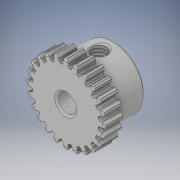
# Autodesk Inventor part: GEABP0.5-24-3-B-3_b
Saved by Autodesk Inventor 2019 (Build 230136000, 136)
## iProperties
Created: 2024-02-14
Part Number: GEABP0.5-24-3-B-3_b
Material: Generic
Catalog Web Link: www.cadenas.de
Description: GEABM, GEABMS, GEABMT, GEABP, GEABPS, GEABPT, GEABA, GEABAS, GEABAT_body-Plastic Spur Gears - Pressure Angle 20 Degrees, Module 0.5/0.8/1.0/1.5/2.0/2.5/3.0
Vendor: MISUMI
Document SubType Name: Modeling
Designer: psAdmin
Manufacturer: MISUMI
Mass: 0.648666 g
Surface Area: 6.64775 cm^2
Volume: 0.648666 cm^3
Density: 1 g/cm^3
Appearance: PSOLRGB-175-175-175
Category: PARTsolutions
Company: MISUMI
Title: GEABP0.5-24-3-B-3
Author: Cadenas PARTsolutions
Comments: Plastic Spur Gears - Pressure Angle 20 Degrees, Module 0.5/0.8/1.0/1.5/2.0/2.5/3.0
PSOL_IDENT_0: {$CADENAS_DATA/23d-libs/misumi/metric/54_spur_gears/geabms20/geabms20.prj},386 {VTYP=3D},{NB=GEABP0.
PSOL_IDENT_1: 5-24-3-B-3_b},{LINA=GEABP0.5-24-3-B-3},{NN=GEABM, GEABMS, GEABMT, GEABP, GEABPS, GEABPT, GEABA, GEAB
PSOL_IDENT_2: AS, GEABAT_body},{DATE=13.11.2023 01:03:00},{GEOMDATE=12.11.2023 05:54:16},{VERSION=},{LINEID=10},{W
PSOL_IDENT_3: BVAR=MATSG,MATCR,NT,B,TS,PS,ALT1,ALT2,TPC,ALT11,ALT10,BS,ALT3,Z,J,ALT4,Q,R,S,T,ALT5,LFC,LTC,MALT5,AL
PSOL_IDENT_4: T6,KFC,KTC,K},{WBNUMERIC=NT,B,BS,Z,J,Q,R,S,T,LFC,LTC,KFC,KTC,K}  {NB=GEABP0.5-24-3-B-3_b},{LINA=GEAB
PSOL_IDENT_5: P0.5-24-3-B-3},{KT=DUMMY},{PN=GEABP0.5-24-3-B-3},{TYPE=GEABP},{MATSG=PW},{MATSGALG='MCN','MC Nylon','
PSOL_IDENT_6: PW','Polyacetal White','PB','Polyacetal Blue'},{MATCR=},{MATCRALG='','-'},{MOD=0.5},{MOD1=0.5},{NT=2
PSOL_IDENT_7: 4},{NTALG=15,16,18,20,24,25,28,30,32,36,40,45,48,50,56,60,64,70,72,80,90,100,120},{B=3},{BALG=3,5},{
PSOL_IDENT_8: TS=B},{TSALG='B','B'},{TSPN=-B},{PS=3},{PSALG='3','3','4','4','5','5','6','6','7','7'},{PSCRL='3','3'
PSOL_IDENT_9: ,'4','4','5','5','6','6','7','7'},{PSCRW='0','0'},{DD=12.0},{DD05=12},{DD08=19.2},{DD10=24},{DD15=36
PSOL_IDENT_10: },{DD20=48},{DD25=60},{DD30=72},{D=13.0},{D05=13},{D08=20.8},{D10=26},{D15=39},{D20=52},{D25=65},{D3
PSOL_IDENT_11: 0=78},{G=10.75},{G05=10.75},{G08=17.2},{G10=21.5},{G15=32.25},{G20=43},{G25=53.75},{G30=64.5},{H=10.
PSOL_IDENT_12: 0},{L=8},{LL1=5},{LL2=2.5},{M=M3},{M3D=3},{P=3.00},{DD1=0},{CIFR=8.8},{CIFM=3},{CIFK=0},{CIFTAP=1},{
PSOL_IDENT_13: ALT1=},{ALT1ALG='','w/o Set Screw','KC90','with KC90 (Set Screw)','KC120','with KC120 (Set Screw)'},
PSOL_IDENT_14: {ALT1PN=},{ALT2=},{ALT2ALG='','w/o TPC (Tapped Hole Dimension)','TPC','with TPC (Tapped Hole Dimensi
PSOL_IDENT_15: on)'},{TPC=N/A},{TPCALG='N/A'},{ALT2PN=},{KC=0},{ALT11=},{ALT11ALG='','Not applicable'},{ALT11PN=},{
PSOL_IDENT_16: DEG=0},{ALT10=},{ALT10ALG= '','w/o BS (Boss Cut)','BS','with BS (Boss Cut)' },{ALT10PN=},{BS=0.0},{B
PSOL_IDENT_17: SALG=0},{BSMIN=6},{BSMINALG=6.000},{BSMAX=5},{LL13D=5},{LL23D=5.5},{LBS=8},{ALT3=},{ALT3ALG= '','w/o
PSOL_IDENT_18: Stepped Hole','DHR','with DHR (Stepped Hole)' },{ALT3PN=},{ZJPN=},{ALT31=0},{ALT32=1},{Z=0},{ZALG=0
PSOL_IDENT_19: },{ZMINL=5},{ZMAXL=6},{ZMINR=5},{ZMAXR=6},{ZPN=},{J=0.0},{JALG=0},{JMIN=2},{JMAX=0},{JPN=},{ALT4=},{
PSOL_IDENT_20: ALT4ALG= '','Not applicable' },{ALT4PN=},{QRSTPN=},{LB=8.000},{Q=0},{QALG=0},{QMIN=5},{QMAX=6},{QPN=
PSOL_IDENT_21: },{R=0},{RALG=0},{RMIN=5},{RMAX=6},{RPN=},{S=0},{SALG=0},{SMIN=3},{SMAX=2},{SPN=},{T=0},{TALG=0},{TM
PSOL_IDENT_22: IN=3},{TMAX=0},{TPN=},{ALT5=},{ALT5ALG= '','Not applicable' },{LFC=0},{LFCALG=0},{LTC=0},{LTCALG=0},
PSOL_IDENT_23: {LPCDMIN=11},{LPCDMAX=3},{LCMAX=6},{MALT5=N/A},{MALT5ALG= 'N/A' },{LCMAX2=3},{C=0.0},{ALT5PN=},{ALT6=
PSOL_IDENT_24: },{ALT6ALG= '','Not applicable' },{ALT6PN=},{KFTCPN=},{KFC=0},{KFCALG=[0]},{KFCPN=},{KTC=0},{KTCALG=
PSOL_IDENT_25: [0]},{KTCPN=},{KPCDMIN1=10},{KPCDMAX1=3},{KPCDMIN2=17},{KPCDMAX2=3},{K=0.0},{KALG=[0]},{KPCD=0},{KPN=
PSOL_IDENT_26: },{SCREW=3},{SCREWL=3},{AG=0},{PCD=0},{SHN=0},{SHDEG1=0},{SHDEG2=0},{PZQRDD2=3},{D1=3.75},{D2=7.5},{
PSOL_IDENT_27: D3=20},{D4=0.05},{D5=2},{D6=1.846154},{D7=0.425},{D8=0.25},{D9=0.408748},{S1=15},{S2=0.5},{KR=8.8}
NB: GEABP0.5-24-3-B-3_b
NN: GEABM, GEABMS, GEABMT, GEABP, GEABPS, GEABPT, GEABA, GEABAS, GEABAT_body
NT: 24
NBSYN: $PN._b
LINA: GEABP0.5-24-3-B-3
CATALOG: Misumi
PN: GEABP0.5-24-3-B-3
MATSG: Polyacetal White
MATCR: -
MOD: 0.5
B: 3
TS: B
PS: 3
DD: 12
D: 13
G: 10.75
H: 10
L: 8
LL1: 5
LL2: 2.5
M: M3
DD1: 0
ALT1: w/o Set Screw
ALT2: w/o TPC (Tapped Hole Dimension)
TPC: N/A
ALT11: Not applicable
ALT10: w/o BS (Boss Cut)
BS: 0
ALT3: w/o Stepped Hole
Z: 0
J: 0
ALT4: Not applicable
Q: 0
R: 0
S: 0
T: 0
ALT5: Not applicable
LFC: 0
LTC: 0
MALT5: N/A
C: 0
ALT6: Not applicable
KFC: 0
KTC: 0
K: 0
SUPPLIER: MISUMI
ARTICLENO: GEABP0.5-24-3-B-3_b
BOMINFO: GEABP0.5-24-3-B-3
CREATOR: CADENAS GmbH
Autodesk Inventor part; units mm, degrees
sketch "Sketch_2" plane through (0, 0, 0) normal (1, 0, 0) x (0, 1, 0)
  line L0 (0, -500) -> (0, 500)
  line L1 (0, 0) -> (6, 0)
  line L2 (6, 0) -> (8.5, -0.6699)
  line L3 (8.5, -0.6699) -> (8.5, -2.3301)
  line L4 (8.5, -2.3301) -> (6, -3)
  line L5 (6, -3) -> (5, -3)
  line L6 (5, -3) -> (5, -7.7)
  line L7 (5, -7.7) -> (4.7, -8)
  line L8 (4.7, -8) -> (0, -8)
  line L9 (0, -8) -> (0, 0)
  constraints: 20 end point
revolve "Revolution1" add sketch "Sketch_2" angle 360 about axis through (0, 0, -500) along (0, 0, -1)
sketch "_____12" plane through (0, 0, 0) normal (0, 0, 1) x (1, 0, 0)
  circle A0 centre (0, 0) radius 26
  arc A1 (-6.4986, 0.1346) -> (-6.4986, -0.1346) centre (0, 0) ccw
  arc A2 (-6.4986, -0.1346) -> (-6.4748, -0.1762) centre (-6.4486, -0.1336) ccw
  arc A3 (-6.4748, -0.1762) -> (-5.9872, -0.3924) centre (-5.4275, 1.5277) ccw
  arc A4 (-5.9872, -0.3924) -> (-5.8765, -0.4087) centre (-5.8728, 0) ccw
  arc A5 (-5.5335, -0.4445) -> (-5.8765, -0.4087) centre (-5.8958, -2.2548) ccw
  arc A6 (-5.3344, -0.659) -> (-5.5335, -0.4445) centre (-5.5826, -0.6897) ccw
  arc A7 (-5.3344, -0.659) -> (-5.3232, -0.7441) centre (0, 0) ccw
  arc A8 (-5.46, -1.0028) -> (-5.3232, -0.7441) centre (-5.5708, -0.7787) ccw
  arc A9 (-5.782, -1.1261) -> (-5.46, -1.0028) centre (-6.2785, 0.652) ccw
  arc A10 (-5.782, -1.1261) -> (-5.8847, -1.1705) centre (-5.6727, -1.52) ccw
  arc A11 (-5.8847, -1.1705) -> (-6.2998, -1.5056) centre (-4.8472, -2.8804) ccw
  arc A12 (-6.2998, -1.5056) -> (-6.312, -1.5519) centre (-6.2635, -1.54) ccw
  arc A13 (-6.312, -1.5519) -> (-6.2423, -1.812) centre (0, 0) ccw
  arc A14 (-6.2423, -1.812) -> (-6.2086, -1.846) centre (-6.1943, -1.7981) ccw
  arc A15 (-6.2086, -1.846) -> (-5.6816, -1.9286) centre (-5.638, 0.0709) ccw
  arc A16 (-5.6816, -1.9286) -> (-5.5704, -1.9157) centre (-5.6727, -1.52) ccw
  arc A17 (-5.2299, -1.8616) -> (-5.5704, -1.9157) centre (-5.1113, -3.7039) ccw
  arc A18 (-4.9821, -2.0172) -> (-5.2299, -1.8616) centre (-5.2138, -2.111) ccw
  arc A19 (-4.9821, -2.0172) -> (-4.9493, -2.0965) centre (0, 0) ccw
  arc A20 (-5.0144, -2.3818) -> (-4.9493, -2.0965) centre (-5.1795, -2.194) ccw
  arc A21 (-5.2935, -2.5843) -> (-5.0144, -2.3818) centre (-6.2333, -0.9952) ccw
  arc A22 (-5.2935, -2.5843) -> (-5.3812, -2.6537) centre (-5.086, -2.9364) ccw
  arc A23 (-5.3812, -2.6537) -> (-5.6954, -3.0848) centre (-3.9365, -4.0368) ccw
  arc A24 (-5.6954, -3.0848) -> (-5.6953, -3.1327) centre (-5.6515, -3.1086) ccw
  arc A25 (-5.6953, -3.1327) -> (-5.5606, -3.3659) centre (0, 0) ccw
  arc A26 (-5.5606, -3.3659) -> (-5.5192, -3.39) centre (-5.5179, -3.34) ccw
  arc A27 (-5.5192, -3.39) -> (-4.9888, -3.3334) centre (-5.4642, -1.3907) ccw
  arc A28 (-4.9888, -3.3334) -> (-4.8848, -3.2922) centre (-5.086, -2.9364) ccw
  arc A29 (-4.5699, -3.1517) -> (-4.8848, -3.2922) centre (-3.9785, -4.9006) ccw
  arc A30 (-4.2903, -3.2379) -> (-4.5699, -3.1517) centre (-4.4898, -3.3885) ccw
  arc A31 (-4.2903, -3.2379) -> (-4.238, -3.306) centre (0, 0) ccw
  arc A32 (-4.2271, -3.5985) -> (-4.238, -3.306) centre (-4.4351, -3.4598) ccw
  arc A33 (-4.4443, -3.8663) -> (-4.2271, -3.5985) centre (-5.7633, -2.5746) ccw
  arc A34 (-4.4443, -3.8663) -> (-4.511, -3.9561) centre (-4.1527, -4.1527) ccw
  arc A35 (-4.511, -3.9561) -> (-4.703, -4.4538) centre (-2.7576, -4.9181) ccw
  arc A36 (-4.703, -4.4538) -> (-4.6904, -4.5) centre (-4.6543, -4.4654) ccw
  arc A37 (-4.6904, -4.5) -> (-4.5, -4.6904) centre (0, 0) ccw
  arc A38 (-4.5, -4.6904) -> (-4.4538, -4.703) centre (-4.4654, -4.6543) ccw
  arc A39 (-4.4538, -4.703) -> (-3.9561, -4.511) centre (-4.9181, -2.7576) ccw
  arc A40 (-3.9561, -4.511) -> (-3.8663, -4.4443) centre (-4.1527, -4.1527) ccw
  arc A41 (-3.5985, -4.2271) -> (-3.8663, -4.4443) centre (-2.5746, -5.7633) ccw
  arc A42 (-3.306, -4.238) -> (-3.5985, -4.2271) centre (-3.4598, -4.4351) ccw
  arc A43 (-3.306, -4.238) -> (-3.2379, -4.2903) centre (0, 0) ccw
  arc A44 (-3.1517, -4.5699) -> (-3.2379, -4.2903) centre (-3.3885, -4.4898) ccw
  arc A45 (-3.2922, -4.8848) -> (-3.1517, -4.5699) centre (-4.9006, -3.9785) ccw
  arc A46 (-3.2922, -4.8848) -> (-3.3334, -4.9888) centre (-2.9364, -5.086) ccw
  arc A47 (-3.3334, -4.9888) -> (-3.39, -5.5192) centre (-1.3907, -5.4642) ccw
  arc A48 (-3.39, -5.5192) -> (-3.3659, -5.5606) centre (-3.34, -5.5179) ccw
  arc A49 (-3.3659, -5.5606) -> (-3.1327, -5.6953) centre (0, 0) ccw
  arc A50 (-3.1327, -5.6953) -> (-3.0848, -5.6954) centre (-3.1086, -5.6515) ccw
  arc A51 (-3.0848, -5.6954) -> (-2.6537, -5.3812) centre (-4.0368, -3.9365) ccw
  arc A52 (-2.6537, -5.3812) -> (-2.5843, -5.2935) centre (-2.9364, -5.086) ccw
  arc A53 (-2.3818, -5.0144) -> (-2.5843, -5.2935) centre (-0.9952, -6.2333) ccw
  arc A54 (-2.0965, -4.9493) -> (-2.3818, -5.0144) centre (-2.194, -5.1795) ccw
  arc A55 (-2.0965, -4.9493) -> (-2.0172, -4.9821) centre (0, 0) ccw
  arc A56 (-1.8616, -5.2299) -> (-2.0172, -4.9821) centre (-2.111, -5.2138) ccw
  arc A57 (-1.9157, -5.5704) -> (-1.8616, -5.2299) centre (-3.7039, -5.1113) ccw
  arc A58 (-1.9157, -5.5704) -> (-1.9286, -5.6816) centre (-1.52, -5.6727) ccw
  arc A59 (-1.9286, -5.6816) -> (-1.846, -6.2086) centre (0.0709, -5.638) ccw
  arc A60 (-1.846, -6.2086) -> (-1.812, -6.2423) centre (-1.7981, -6.1943) ccw
  arc A61 (-1.812, -6.2423) -> (-1.5519, -6.312) centre (0, 0) ccw
  arc A62 (-1.5519, -6.312) -> (-1.5056, -6.2998) centre (-1.54, -6.2635) ccw
  arc A63 (-1.5056, -6.2998) -> (-1.1705, -5.8847) centre (-2.8804, -4.8472) ccw
  arc A64 (-1.1705, -5.8847) -> (-1.1261, -5.782) centre (-1.52, -5.6727) ccw
  arc A65 (-1.0028, -5.46) -> (-1.1261, -5.782) centre (0.652, -6.2785) ccw
  arc A66 (-0.7441, -5.3232) -> (-1.0028, -5.46) centre (-0.7787, -5.5708) ccw
  arc A67 (-0.7441, -5.3232) -> (-0.659, -5.3344) centre (0, 0) ccw
  arc A68 (-0.4445, -5.5335) -> (-0.659, -5.3344) centre (-0.6897, -5.5826) ccw
  arc A69 (-0.4087, -5.8765) -> (-0.4445, -5.5335) centre (-2.2548, -5.8958) ccw
  arc A70 (-0.4087, -5.8765) -> (-0.3924, -5.9872) centre (0, -5.8728) ccw
  arc A71 (-0.3924, -5.9872) -> (-0.1762, -6.4748) centre (1.5277, -5.4275) ccw
  arc A72 (-0.1762, -6.4748) -> (-0.1346, -6.4986) centre (-0.1336, -6.4486) ccw
  arc A73 (-0.1346, -6.4986) -> (0.1346, -6.4986) centre (0, 0) ccw
  arc A74 (0.1346, -6.4986) -> (0.1762, -6.4748) centre (0.1336, -6.4486) ccw
  arc A75 (0.1762, -6.4748) -> (0.3924, -5.9872) centre (-1.5277, -5.4275) ccw
  arc A76 (0.3924, -5.9872) -> (0.4087, -5.8765) centre (0, -5.8728) ccw
  arc A77 (0.4445, -5.5335) -> (0.4087, -5.8765) centre (2.2548, -5.8958) ccw
  arc A78 (0.659, -5.3344) -> (0.4445, -5.5335) centre (0.6897, -5.5826) ccw
  arc A79 (0.659, -5.3344) -> (0.7441, -5.3232) centre (0, 0) ccw
  arc A80 (1.0028, -5.46) -> (0.7441, -5.3232) centre (0.7787, -5.5708) ccw
  arc A81 (1.1261, -5.782) -> (1.0028, -5.46) centre (-0.652, -6.2785) ccw
  arc A82 (1.1261, -5.782) -> (1.1705, -5.8847) centre (1.52, -5.6727) ccw
  arc A83 (1.1705, -5.8847) -> (1.5056, -6.2998) centre (2.8804, -4.8472) ccw
  arc A84 (1.5056, -6.2998) -> (1.5519, -6.312) centre (1.54, -6.2635) ccw
  arc A85 (1.5519, -6.312) -> (1.812, -6.2423) centre (0, 0) ccw
  arc A86 (1.812, -6.2423) -> (1.846, -6.2086) centre (1.7981, -6.1943) ccw
  arc A87 (1.846, -6.2086) -> (1.9286, -5.6816) centre (-0.0709, -5.638) ccw
  arc A88 (1.9286, -5.6816) -> (1.9157, -5.5704) centre (1.52, -5.6727) ccw
  arc A89 (1.8616, -5.2299) -> (1.9157, -5.5704) centre (3.7039, -5.1113) ccw
  arc A90 (2.0172, -4.9821) -> (1.8616, -5.2299) centre (2.111, -5.2138) ccw
  arc A91 (2.0172, -4.9821) -> (2.0965, -4.9493) centre (0, 0) ccw
  arc A92 (2.3818, -5.0144) -> (2.0965, -4.9493) centre (2.194, -5.1795) ccw
  arc A93 (2.5843, -5.2935) -> (2.3818, -5.0144) centre (0.9952, -6.2333) ccw
  arc A94 (2.5843, -5.2935) -> (2.6537, -5.3812) centre (2.9364, -5.086) ccw
  arc A95 (2.6537, -5.3812) -> (3.0848, -5.6954) centre (4.0368, -3.9365) ccw
  arc A96 (3.0848, -5.6954) -> (3.1327, -5.6953) centre (3.1086, -5.6515) ccw
  arc A97 (3.1327, -5.6953) -> (3.3659, -5.5606) centre (0, 0) ccw
  arc A98 (3.3659, -5.5606) -> (3.39, -5.5192) centre (3.34, -5.5179) ccw
  arc A99 (3.39, -5.5192) -> (3.3334, -4.9888) centre (1.3907, -5.4642) ccw
  arc A100 (3.3334, -4.9888) -> (3.2922, -4.8848) centre (2.9364, -5.086) ccw
  arc A101 (3.1517, -4.5699) -> (3.2922, -4.8848) centre (4.9006, -3.9785) ccw
  arc A102 (3.2379, -4.2903) -> (3.1517, -4.5699) centre (3.3885, -4.4898) ccw
  arc A103 (3.2379, -4.2903) -> (3.306, -4.238) centre (0, 0) ccw
  arc A104 (3.5985, -4.2271) -> (3.306, -4.238) centre (3.4598, -4.4351) ccw
  arc A105 (3.8663, -4.4443) -> (3.5985, -4.2271) centre (2.5746, -5.7633) ccw
  arc A106 (3.8663, -4.4443) -> (3.9561, -4.511) centre (4.1527, -4.1527) ccw
  arc A107 (3.9561, -4.511) -> (4.4538, -4.703) centre (4.9181, -2.7576) ccw
  arc A108 (4.4538, -4.703) -> (4.5, -4.6904) centre (4.4654, -4.6543) ccw
  arc A109 (4.5, -4.6904) -> (4.6904, -4.5) centre (0, 0) ccw
  arc A110 (4.6904, -4.5) -> (4.703, -4.4538) centre (4.6543, -4.4654) ccw
  arc A111 (4.703, -4.4538) -> (4.511, -3.9561) centre (2.7576, -4.9181) ccw
  arc A112 (4.511, -3.9561) -> (4.4443, -3.8663) centre (4.1527, -4.1527) ccw
  arc A113 (4.2271, -3.5985) -> (4.4443, -3.8663) centre (5.7633, -2.5746) ccw
  arc A114 (4.238, -3.306) -> (4.2271, -3.5985) centre (4.4351, -3.4598) ccw
  arc A115 (4.238, -3.306) -> (4.2903, -3.2379) centre (0, 0) ccw
  arc A116 (4.5699, -3.1517) -> (4.2903, -3.2379) centre (4.4898, -3.3885) ccw
  arc A117 (4.8848, -3.2922) -> (4.5699, -3.1517) centre (3.9785, -4.9006) ccw
  arc A118 (4.8848, -3.2922) -> (4.9888, -3.3334) centre (5.086, -2.9364) ccw
  arc A119 (4.9888, -3.3334) -> (5.5192, -3.39) centre (5.4642, -1.3907) ccw
  arc A120 (5.5192, -3.39) -> (5.5606, -3.3659) centre (5.5179, -3.34) ccw
  arc A121 (5.5606, -3.3659) -> (5.6953, -3.1327) centre (0, 0) ccw
  arc A122 (5.6953, -3.1327) -> (5.6954, -3.0848) centre (5.6515, -3.1086) ccw
  arc A123 (5.6954, -3.0848) -> (5.3812, -2.6537) centre (3.9365, -4.0368) ccw
  arc A124 (5.3812, -2.6537) -> (5.2935, -2.5843) centre (5.086, -2.9364) ccw
  arc A125 (5.0144, -2.3818) -> (5.2935, -2.5843) centre (6.2333, -0.9952) ccw
  arc A126 (4.9493, -2.0965) -> (5.0144, -2.3818) centre (5.1795, -2.194) ccw
  arc A127 (4.9493, -2.0965) -> (4.9821, -2.0172) centre (0, 0) ccw
  arc A128 (5.2299, -1.8616) -> (4.9821, -2.0172) centre (5.2138, -2.111) ccw
  arc A129 (5.5704, -1.9157) -> (5.2299, -1.8616) centre (5.1113, -3.7039) ccw
  arc A130 (5.5704, -1.9157) -> (5.6816, -1.9286) centre (5.6727, -1.52) ccw
  arc A131 (5.6816, -1.9286) -> (6.2086, -1.846) centre (5.638, 0.0709) ccw
  arc A132 (6.2086, -1.846) -> (6.2423, -1.812) centre (6.1943, -1.7981) ccw
  arc A133 (6.2423, -1.812) -> (6.312, -1.5519) centre (0, 0) ccw
  arc A134 (6.312, -1.5519) -> (6.2998, -1.5056) centre (6.2635, -1.54) ccw
  arc A135 (6.2998, -1.5056) -> (5.8847, -1.1705) centre (4.8472, -2.8804) ccw
  arc A136 (5.8847, -1.1705) -> (5.782, -1.1261) centre (5.6727, -1.52) ccw
  arc A137 (5.46, -1.0028) -> (5.782, -1.1261) centre (6.2785, 0.652) ccw
  arc A138 (5.3232, -0.7441) -> (5.46, -1.0028) centre (5.5708, -0.7787) ccw
  arc A139 (5.3232, -0.7441) -> (5.3344, -0.659) centre (0, 0) ccw
  arc A140 (5.5335, -0.4445) -> (5.3344, -0.659) centre (5.5826, -0.6897) ccw
  arc A141 (5.8765, -0.4087) -> (5.5335, -0.4445) centre (5.8958, -2.2548) ccw
  arc A142 (5.8765, -0.4087) -> (5.9872, -0.3924) centre (5.8728, 0) ccw
  arc A143 (5.9872, -0.3924) -> (6.4748, -0.1762) centre (5.4275, 1.5277) ccw
  arc A144 (6.4748, -0.1762) -> (6.4986, -0.1346) centre (6.4486, -0.1336) ccw
  arc A145 (6.4986, -0.1346) -> (6.4986, 0.1346) centre (0, 0) ccw
  arc A146 (6.4986, 0.1346) -> (6.4748, 0.1762) centre (6.4486, 0.1336) ccw
  arc A147 (6.4748, 0.1762) -> (5.9872, 0.3924) centre (5.4275, -1.5277) ccw
  arc A148 (5.9872, 0.3924) -> (5.8765, 0.4087) centre (5.8728, 0) ccw
  arc A149 (5.5335, 0.4445) -> (5.8765, 0.4087) centre (5.8958, 2.2548) ccw
  arc A150 (5.3344, 0.659) -> (5.5335, 0.4445) centre (5.5826, 0.6897) ccw
  arc A151 (5.3344, 0.659) -> (5.3232, 0.7441) centre (0, 0) ccw
  arc A152 (5.46, 1.0028) -> (5.3232, 0.7441) centre (5.5708, 0.7787) ccw
  arc A153 (5.782, 1.1261) -> (5.46, 1.0028) centre (6.2785, -0.652) ccw
  arc A154 (5.782, 1.1261) -> (5.8847, 1.1705) centre (5.6727, 1.52) ccw
  arc A155 (5.8847, 1.1705) -> (6.2998, 1.5056) centre (4.8472, 2.8804) ccw
  arc A156 (6.2998, 1.5056) -> (6.312, 1.5519) centre (6.2635, 1.54) ccw
  arc A157 (6.312, 1.5519) -> (6.2423, 1.812) centre (0, 0) ccw
  arc A158 (6.2423, 1.812) -> (6.2086, 1.846) centre (6.1943, 1.7981) ccw
  arc A159 (6.2086, 1.846) -> (5.6816, 1.9286) centre (5.638, -0.0709) ccw
  arc A160 (5.6816, 1.9286) -> (5.5704, 1.9157) centre (5.6727, 1.52) ccw
  arc A161 (5.2299, 1.8616) -> (5.5704, 1.9157) centre (5.1113, 3.7039) ccw
  arc A162 (4.9821, 2.0172) -> (5.2299, 1.8616) centre (5.2138, 2.111) ccw
  arc A163 (4.9821, 2.0172) -> (4.9493, 2.0965) centre (0, 0) ccw
  arc A164 (5.0144, 2.3818) -> (4.9493, 2.0965) centre (5.1795, 2.194) ccw
  arc A165 (5.2935, 2.5843) -> (5.0144, 2.3818) centre (6.2333, 0.9952) ccw
  arc A166 (5.2935, 2.5843) -> (5.3812, 2.6537) centre (5.086, 2.9364) ccw
  arc A167 (5.3812, 2.6537) -> (5.6954, 3.0848) centre (3.9365, 4.0368) ccw
  arc A168 (5.6954, 3.0848) -> (5.6953, 3.1327) centre (5.6515, 3.1086) ccw
  arc A169 (5.6953, 3.1327) -> (5.5606, 3.3659) centre (0, 0) ccw
  arc A170 (5.5606, 3.3659) -> (5.5192, 3.39) centre (5.5179, 3.34) ccw
  arc A171 (5.5192, 3.39) -> (4.9888, 3.3334) centre (5.4642, 1.3907) ccw
  arc A172 (4.9888, 3.3334) -> (4.8848, 3.2922) centre (5.086, 2.9364) ccw
  arc A173 (4.5699, 3.1517) -> (4.8848, 3.2922) centre (3.9785, 4.9006) ccw
  arc A174 (4.2903, 3.2379) -> (4.5699, 3.1517) centre (4.4898, 3.3885) ccw
  arc A175 (4.2903, 3.2379) -> (4.238, 3.306) centre (0, 0) ccw
  arc A176 (4.2271, 3.5985) -> (4.238, 3.306) centre (4.4351, 3.4598) ccw
  arc A177 (4.4443, 3.8663) -> (4.2271, 3.5985) centre (5.7633, 2.5746) ccw
  arc A178 (4.4443, 3.8663) -> (4.511, 3.9561) centre (4.1527, 4.1527) ccw
  arc A179 (4.511, 3.9561) -> (4.703, 4.4538) centre (2.7576, 4.9181) ccw
  arc A180 (4.703, 4.4538) -> (4.6904, 4.5) centre (4.6543, 4.4654) ccw
  arc A181 (4.6904, 4.5) -> (4.5, 4.6904) centre (0, 0) ccw
  arc A182 (4.5, 4.6904) -> (4.4538, 4.703) centre (4.4654, 4.6543) ccw
  arc A183 (4.4538, 4.703) -> (3.9561, 4.511) centre (4.9181, 2.7576) ccw
  arc A184 (3.9561, 4.511) -> (3.8663, 4.4443) centre (4.1527, 4.1527) ccw
  arc A185 (3.5985, 4.2271) -> (3.8663, 4.4443) centre (2.5746, 5.7633) ccw
  arc A186 (3.306, 4.238) -> (3.5985, 4.2271) centre (3.4598, 4.4351) ccw
  arc A187 (3.306, 4.238) -> (3.2379, 4.2903) centre (0, 0) ccw
  arc A188 (3.1517, 4.5699) -> (3.2379, 4.2903) centre (3.3885, 4.4898) ccw
  arc A189 (3.2922, 4.8848) -> (3.1517, 4.5699) centre (4.9006, 3.9785) ccw
  arc A190 (3.2922, 4.8848) -> (3.3334, 4.9888) centre (2.9364, 5.086) ccw
  arc A191 (3.3334, 4.9888) -> (3.39, 5.5192) centre (1.3907, 5.4642) ccw
  arc A192 (3.39, 5.5192) -> (3.3659, 5.5606) centre (3.34, 5.5179) ccw
  arc A193 (3.3659, 5.5606) -> (3.1327, 5.6953) centre (0, 0) ccw
  arc A194 (3.1327, 5.6953) -> (3.0848, 5.6954) centre (3.1086, 5.6515) ccw
  arc A195 (3.0848, 5.6954) -> (2.6537, 5.3812) centre (4.0368, 3.9365) ccw
  arc A196 (2.6537, 5.3812) -> (2.5843, 5.2935) centre (2.9364, 5.086) ccw
  arc A197 (2.3818, 5.0144) -> (2.5843, 5.2935) centre (0.9952, 6.2333) ccw
  arc A198 (2.0965, 4.9493) -> (2.3818, 5.0144) centre (2.194, 5.1795) ccw
  arc A199 (2.0965, 4.9493) -> (2.0172, 4.9821) centre (0, 0) ccw
  arc A200 (1.8616, 5.2299) -> (2.0172, 4.9821) centre (2.111, 5.2138) ccw
  arc A201 (1.9157, 5.5704) -> (1.8616, 5.2299) centre (3.7039, 5.1113) ccw
  arc A202 (1.9157, 5.5704) -> (1.9286, 5.6816) centre (1.52, 5.6727) ccw
  arc A203 (1.9286, 5.6816) -> (1.846, 6.2086) centre (-0.0709, 5.638) ccw
  arc A204 (1.846, 6.2086) -> (1.812, 6.2423) centre (1.7981, 6.1943) ccw
  arc A205 (1.812, 6.2423) -> (1.5519, 6.312) centre (0, 0) ccw
  arc A206 (1.5519, 6.312) -> (1.5056, 6.2998) centre (1.54, 6.2635) ccw
  arc A207 (1.5056, 6.2998) -> (1.1705, 5.8847) centre (2.8804, 4.8472) ccw
  arc A208 (1.1705, 5.8847) -> (1.1261, 5.782) centre (1.52, 5.6727) ccw
  arc A209 (1.0028, 5.46) -> (1.1261, 5.782) centre (-0.652, 6.2785) ccw
  arc A210 (0.7441, 5.3232) -> (1.0028, 5.46) centre (0.7787, 5.5708) ccw
  arc A211 (0.7441, 5.3232) -> (0.659, 5.3344) centre (0, 0) ccw
  arc A212 (0.4445, 5.5335) -> (0.659, 5.3344) centre (0.6897, 5.5826) ccw
  arc A213 (0.4087, 5.8765) -> (0.4445, 5.5335) centre (2.2548, 5.8958) ccw
  arc A214 (0.4087, 5.8765) -> (0.3924, 5.9872) centre (0, 5.8728) ccw
  arc A215 (0.3924, 5.9872) -> (0.1762, 6.4748) centre (-1.5277, 5.4275) ccw
  arc A216 (0.1762, 6.4748) -> (0.1346, 6.4986) centre (0.1336, 6.4486) ccw
  arc A217 (0.1346, 6.4986) -> (-0.1346, 6.4986) centre (0, 0) ccw
  arc A218 (-0.1346, 6.4986) -> (-0.1762, 6.4748) centre (-0.1336, 6.4486) ccw
  arc A219 (-0.1762, 6.4748) -> (-0.3924, 5.9872) centre (1.5277, 5.4275) ccw
  arc A220 (-0.3924, 5.9872) -> (-0.4087, 5.8765) centre (0, 5.8728) ccw
  arc A221 (-0.4445, 5.5335) -> (-0.4087, 5.8765) centre (-2.2548, 5.8958) ccw
  arc A222 (-0.659, 5.3344) -> (-0.4445, 5.5335) centre (-0.6897, 5.5826) ccw
  arc A223 (-0.659, 5.3344) -> (-0.7441, 5.3232) centre (0, 0) ccw
  arc A224 (-1.0028, 5.46) -> (-0.7441, 5.3232) centre (-0.7787, 5.5708) ccw
  arc A225 (-1.1261, 5.782) -> (-1.0028, 5.46) centre (0.652, 6.2785) ccw
  arc A226 (-1.1261, 5.782) -> (-1.1705, 5.8847) centre (-1.52, 5.6727) ccw
  arc A227 (-1.1705, 5.8847) -> (-1.5056, 6.2998) centre (-2.8804, 4.8472) ccw
  arc A228 (-1.5056, 6.2998) -> (-1.5519, 6.312) centre (-1.54, 6.2635) ccw
  arc A229 (-1.5519, 6.312) -> (-1.812, 6.2423) centre (0, 0) ccw
  arc A230 (-1.812, 6.2423) -> (-1.846, 6.2086) centre (-1.7981, 6.1943) ccw
  arc A231 (-1.846, 6.2086) -> (-1.9286, 5.6816) centre (0.0709, 5.638) ccw
  arc A232 (-1.9286, 5.6816) -> (-1.9157, 5.5704) centre (-1.52, 5.6727) ccw
  arc A233 (-1.8616, 5.2299) -> (-1.9157, 5.5704) centre (-3.7039, 5.1113) ccw
  arc A234 (-2.0172, 4.9821) -> (-1.8616, 5.2299) centre (-2.111, 5.2138) ccw
  arc A235 (-2.0172, 4.9821) -> (-2.0965, 4.9493) centre (0, 0) ccw
  arc A236 (-2.3818, 5.0144) -> (-2.0965, 4.9493) centre (-2.194, 5.1795) ccw
  arc A237 (-2.5843, 5.2935) -> (-2.3818, 5.0144) centre (-0.9952, 6.2333) ccw
  arc A238 (-2.5843, 5.2935) -> (-2.6537, 5.3812) centre (-2.9364, 5.086) ccw
  arc A239 (-2.6537, 5.3812) -> (-3.0848, 5.6954) centre (-4.0368, 3.9365) ccw
  arc A240 (-3.0848, 5.6954) -> (-3.1327, 5.6953) centre (-3.1086, 5.6515) ccw
  arc A241 (-3.1327, 5.6953) -> (-3.3659, 5.5606) centre (0, 0) ccw
  arc A242 (-3.3659, 5.5606) -> (-3.39, 5.5192) centre (-3.34, 5.5179) ccw
  arc A243 (-3.39, 5.5192) -> (-3.3334, 4.9888) centre (-1.3907, 5.4642) ccw
  arc A244 (-3.3334, 4.9888) -> (-3.2922, 4.8848) centre (-2.9364, 5.086) ccw
  arc A245 (-3.1517, 4.5699) -> (-3.2922, 4.8848) centre (-4.9006, 3.9785) ccw
  arc A246 (-3.2379, 4.2903) -> (-3.1517, 4.5699) centre (-3.3885, 4.4898) ccw
  arc A247 (-3.2379, 4.2903) -> (-3.306, 4.238) centre (0, 0) ccw
  arc A248 (-3.5985, 4.2271) -> (-3.306, 4.238) centre (-3.4598, 4.4351) ccw
  arc A249 (-3.8663, 4.4443) -> (-3.5985, 4.2271) centre (-2.5746, 5.7633) ccw
  arc A250 (-3.8663, 4.4443) -> (-3.9561, 4.511) centre (-4.1527, 4.1527) ccw
  arc A251 (-3.9561, 4.511) -> (-4.4538, 4.703) centre (-4.9181, 2.7576) ccw
  arc A252 (-4.4538, 4.703) -> (-4.5, 4.6904) centre (-4.4654, 4.6543) ccw
  arc A253 (-4.5, 4.6904) -> (-4.6904, 4.5) centre (0, 0) ccw
  arc A254 (-4.6904, 4.5) -> (-4.703, 4.4538) centre (-4.6543, 4.4654) ccw
  arc A255 (-4.703, 4.4538) -> (-4.511, 3.9561) centre (-2.7576, 4.9181) ccw
  arc A256 (-4.511, 3.9561) -> (-4.4443, 3.8663) centre (-4.1527, 4.1527) ccw
  arc A257 (-4.2271, 3.5985) -> (-4.4443, 3.8663) centre (-5.7633, 2.5746) ccw
  arc A258 (-4.238, 3.306) -> (-4.2271, 3.5985) centre (-4.4351, 3.4598) ccw
  arc A259 (-4.238, 3.306) -> (-4.2903, 3.2379) centre (0, 0) ccw
  arc A260 (-4.5699, 3.1517) -> (-4.2903, 3.2379) centre (-4.4898, 3.3885) ccw
  arc A261 (-4.8848, 3.2922) -> (-4.5699, 3.1517) centre (-3.9785, 4.9006) ccw
  arc A262 (-4.8848, 3.2922) -> (-4.9888, 3.3334) centre (-5.086, 2.9364) ccw
  arc A263 (-4.9888, 3.3334) -> (-5.5192, 3.39) centre (-5.4642, 1.3907) ccw
  arc A264 (-5.5192, 3.39) -> (-5.5606, 3.3659) centre (-5.5179, 3.34) ccw
  arc A265 (-5.5606, 3.3659) -> (-5.6953, 3.1327) centre (0, 0) ccw
  arc A266 (-5.6953, 3.1327) -> (-5.6954, 3.0848) centre (-5.6515, 3.1086) ccw
  arc A267 (-5.6954, 3.0848) -> (-5.3812, 2.6537) centre (-3.9365, 4.0368) ccw
  arc A268 (-5.3812, 2.6537) -> (-5.2935, 2.5843) centre (-5.086, 2.9364) ccw
  arc A269 (-5.0144, 2.3818) -> (-5.2935, 2.5843) centre (-6.2333, 0.9952) ccw
  arc A270 (-4.9493, 2.0965) -> (-5.0144, 2.3818) centre (-5.1795, 2.194) ccw
  arc A271 (-4.9493, 2.0965) -> (-4.9821, 2.0172) centre (0, 0) ccw
  arc A272 (-5.2299, 1.8616) -> (-4.9821, 2.0172) centre (-5.2138, 2.111) ccw
  arc A273 (-5.5704, 1.9157) -> (-5.2299, 1.8616) centre (-5.1113, 3.7039) ccw
  arc A274 (-5.5704, 1.9157) -> (-5.6816, 1.9286) centre (-5.6727, 1.52) ccw
  arc A275 (-5.6816, 1.9286) -> (-6.2086, 1.846) centre (-5.638, -0.0709) ccw
  arc A276 (-6.2086, 1.846) -> (-6.2423, 1.812) centre (-6.1943, 1.7981) ccw
  arc A277 (-6.2423, 1.812) -> (-6.312, 1.5519) centre (0, 0) ccw
  arc A278 (-6.312, 1.5519) -> (-6.2998, 1.5056) centre (-6.2635, 1.54) ccw
  arc A279 (-6.2998, 1.5056) -> (-5.8847, 1.1705) centre (-4.8472, 2.8804) ccw
  arc A280 (-5.8847, 1.1705) -> (-5.782, 1.1261) centre (-5.6727, 1.52) ccw
  arc A281 (-5.46, 1.0028) -> (-5.782, 1.1261) centre (-6.2785, -0.652) ccw
  arc A282 (-5.3232, 0.7441) -> (-5.46, 1.0028) centre (-5.5708, 0.7787) ccw
  arc A283 (-5.3232, 0.7441) -> (-5.3344, 0.659) centre (0, 0) ccw
  arc A284 (-5.5335, 0.4445) -> (-5.3344, 0.659) centre (-5.5826, 0.6897) ccw
  arc A285 (-5.8765, 0.4087) -> (-5.5335, 0.4445) centre (-5.8958, 2.2548) ccw
  arc A286 (-5.8765, 0.4087) -> (-5.9872, 0.3924) centre (-5.8728, 0) ccw
  arc A287 (-5.9872, 0.3924) -> (-6.4748, 0.1762) centre (-5.4275, -1.5277) ccw
  arc A288 (-6.4748, 0.1762) -> (-6.4986, 0.1346) centre (-6.4486, 0.1336) ccw
  constraints: 576 point on circle, 289 centre point
extrude "Extrusion1" cut sketch "_____12" against normal blind 3
sketch "Sketch3" plane through (0, 0, -8) normal (0, 0, -1) x (-1, 0, 0)
  point P0 (0, 0)
hole "Hole1" at (0, 0, -8) direction (0, 0, 1) diameter 3 depth 8
sketch "_____5" plane through (0, 0, 0) normal (1, 0, 0) x (0, 0, -1)
  line L0 (500, 0) -> (-500, 0)
  line L1 (7.7, 1.5) -> (8, 1.5)
  line L2 (8, 1.5) -> (8, 1.8)
  line L3 (8, 1.8) -> (7.7, 1.5)
  constraints: 8 end point
revolve "Revolution2" cut sketch "_____5" angle 360 about axis through (0, 0, -500) along (0, 0, -1)
sketch "_____13" plane through (0, 0, 0) normal (1, 0, 0) x (0, 0, -1)
  line L0 (500, 0) -> (-500, 0)
  line L1 (0, 1.8) -> (0, 1.5)
  line L2 (0, 1.5) -> (0.3, 1.5)
  line L3 (0.3, 1.5) -> (0, 1.8)
  constraints: 8 end point
revolve "Revolution3" cut sketch "_____13" angle 360 about axis through (0, 0, -500) along (0, 0, -1)
sketch "Sketch_4" plane through (0, 0, -5.5) normal (0, 0, 1) x (1, 0, 0)
  line L0 (0, 5) -> (0, 0)
  line L1 (0, 0) -> (-1.2295, 0)
  line L2 (-1.2295, 0) -> (-1.2295, 4.7295)
  line L3 (-1.2295, 4.7295) -> (-1.5, 5)
  line L4 (-1.5, 5) -> (0, 5)
  line L5 (0, 5) -> (0, 0)
  constraints: 12 end point
revolve "Revolution4" cut sketch "Sketch_4" angle 360 about axis through (0, 5, -5.5) along (0, 1, 0)
thread "Thread1" size "M3x0.5" class "6H" standard "ISO Metric profile" length 3.2295
ref_plane "gear_to_screw_XY" through (0, 1.5, -5.5) normal (0, 1, 0) x (1, 0, 0)
ref_plane "gear_to_screw_YZ" through (0, 1.5, -5.5) normal (1, 0, 0) x (0, 0, -1)
ref_plane "gear_to_screw_ZX" through (0, 1.5, -5.5) normal (0, 0, -1) x (0, 1, 0)
body "Solid1"
